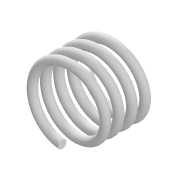
# Autodesk Inventor part: 弹簧
Saved by Autodesk Inventor 2022 (Build 260153000, 153)
## iProperties
Created: 2023-03-15
Part Number: 弹簧
Material: 常规
Document SubType Name: Modeling
Designer: Lzy18
Density: 1 g/cm^3
Appearance: 默认
Author: Lzy18
Autodesk Inventor part; units mm, degrees
ref_plane "YZ Plane" through (0, 0, 0) normal (1, 0, 0) x (0, 1, 0)
ref_plane "XZ Plane" through (0, 0, 0) normal (0, 1, 0) x (-1, 0, 0)
ref_plane "XY Plane" through (0, 0, 0) normal (0, 0, 1) x (1, 0, 0)
sketch "草图1" plane through (0, 0, 0) normal (1, 0, 0) x (0, 1, 0)
  line L0 (40.3488, 3) -> (-41.6512, 3) projected
  line L1 (26.8219, 33.5) -> (84.8219, 33.5) projected
  line L2 (22.8349, 0) -> (-22.8349, 0) projected
  circle A0 centre (-20, 31) radius 2.5
  line L3 (0, 33.5) -> (0, 0)
  dimension "d0" = 33.5
  dimension "d1" = 5
  dimension "d2" = 20
  constraints: 2 end point, 1 centre point, 1 point on line, 1 tangent, 1 vertical
  measures "d0" distance between parallel lines of L1 L2
  measures "d1" diameter of A0
  measures "d2" distance from line of L3 A0.centre
coil "螺旋扫掠1" sketch "草图1" operation add axis through (0, 0, 33.5) along (0, 0, -1) pitch 8 turns 4.1875 hand right
